L3 (Autodesk Fusion 360 design; units mm, degrees)
part number: 2026-06-01-06-58-29-106
Autodesk Fusion 360 part; units mm, degrees
sketch "Sketch1" plane through (0, 0, 0) normal (0, 0, 1) x (1, 0, 0)
  circle A0 centre (15, 20) radius 4.25
  circle A1 centre (15, 20) radius 2.75
  dimension "d1" = 8.5
  dimension "d2" = 5.5
  constraint concentric A0 A1
  measures "d1" diameter of A0
  measures "d2" diameter of A1
sketch "Sketch2" plane through (0, 0, 0) normal (0, 1, 0) x (1, 0, 0)
  circle A0 centre (0, 0) radius 2.75
  circle A1 centre (0, 0) radius 4.25
  dimension "d5" = 5.5
  dimension "d6" = 8.5
  constraint coincident A0.centre A1.centre
  measures "d5" diameter of A0
  measures "d6" diameter of A1
extrude "Extrude2" add sketch "Sketch2" along normal blind 10
sketch "Sketch3" plane through (0, 0, 0) normal (0, 1, 0) x (1, 0, 0)
sketch "Sketch4" plane through (0, 0, 0) normal (1, 0, 0) x (0, 1, 0)
  line L0 (3, 4.25) -> (7, 4.25)
  line L1 (7, 4.25) -> (7, 3.25)
  line L2 (7, 3.25) -> (3, 3.25)
  line L3 (3, 4.25) -> (3, 3.25)
  line L4 (7, -3.2534) -> (7, -4.2534)
  line L5 (7, -4.2534) -> (3, -4.2534)
  line L6 (3, -4.2534) -> (3, -3.2534)
  line L7 (3, -3.2534) -> (7, -3.2534)
  line L8 (3, -4.2534) -> (3, -3.2534)
  line L9 (3, 3.25) -> (3, 4.25)
  dimension "d9" = 1
  dimension "d10" = 1
  constraint horizontal L0
  constraint perpendicular L0 L1
  constraint perpendicular L1 L2
  constraint perpendicular L2 L4
  constraint perpendicular L3 L5
  constraint perpendicular L0 L9
  constraint perpendicular L5 L6
  constraint perpendicular L4 L7
  constraint collinear L8 L9
  measures "d9" distance of L0.end L1.end
  measures "d10" distance of L5.end L6.end
